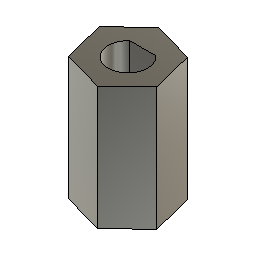
4_Assembly_Wheel - Center - Left v19 (Autodesk Fusion 360 archive; units mm, degrees)
design "Moyeu 18mm"
Autodesk Fusion 360 part; units mm, degrees
note: some values were not read from the file. Chosen so that the rebuilt part matches the saved one: a direction; which face or edge a step refers to. Set by a fixed rule: which sketch regions a step uses.
sketch "Sketch1" plane through (0, 0, 0) normal (0, 0, 1) x (1, 0, 0)
  line L0 (6.5544, -1.8584) -> (4.8866, 4.747)
  line L1 (4.8866, 4.747) -> (-1.6677, 6.6055)
  line L2 (-1.6677, 6.6055) -> (-6.5544, 1.8584)
  line L3 (-6.5544, 1.8584) -> (-4.8866, -4.747)
  line L4 (-4.8866, -4.747) -> (1.6677, -6.6055)
  line L5 (1.6677, -6.6055) -> (6.5544, -1.8584)
  circle A0 centre (0, 0) radius 5
  circle A1 centre (0, 0) radius 3.2
  line L6 (-2.1166, 2.4) -> (2.1166, 2.4)
  line L7 (0, -3.2) -> (9, -3.2) construction
  dimension "d1" = 11.8
  dimension "d2" = 10
  dimension "d7" = 6.4
  dimension "d10" = 5.6
  constraint coincident A0.centre A1.centre
  constraint coincident A1 L6.start
  constraint coincident A1 L6.end
  constraint horizontal L6
  constraint coincident A1 L7.start
  constraint tangent A1 L7
  constraint horizontal L7
  measures "d1" distance of L2 L5
  measures "d2" diameter of A0
  measures "d7" diameter of A1
  measures "d10" distance of L6 L7.start
extrude "Extrude1" add sketch "Sketch1" along normal blind 20 contours A0 | A1 L6 picked at (-0.1815, 2.7157)
extrude "Extrude2" add sketch "Sketch1" along normal blind 20 contours L0 L1 L2 L3 L4 L5

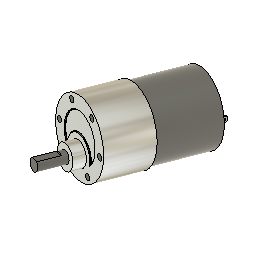
design "Moteur D37"
Autodesk Fusion 360 part; units mm, degrees
sketch "Sketch1" plane through (0, 0, 0) normal (0, 0, 1) x (1, 0, 0)
  circle A0 centre (0, 0) radius 17.4
  dimension "d2" = 34.8
  measures "d2" diameter of A0
extrude "Extrude2" add sketch "Sketch1" along normal blind 30.7
sketch "Sketch2" plane through (0, 0, 30.7) normal (0, 0, 1) x (-1, 0, 0)
  circle A0 centre (0, 0) radius 17.4
  circle A1 centre (0, 0) radius 18.4
  dimension "d7" = 36.8
  constraint coincident A0.centre A1.centre
  measures "d7" diameter of A1
extrude "Extrude3" add sketch "Sketch2" along normal blind 24 contours A0 | A1
sketch "Sketch3" plane through (0, 0, 54.7) normal (0, 0, 1) x (-1, 0, 0)
  circle A0 centre (0, 0) radius 18.4
  circle A1 centre (0, 7) radius 6
  circle A2 centre (0, 7) radius 3
  circle A3 centre (15.5, 0) radius 1.5
  circle A4 centre (7.75, -13.4234) radius 1.5
  circle A5 centre (-7.75, -13.4234) radius 1.5
  circle A6 centre (-15.5, 0) radius 1.5
  circle A7 centre (7.75, 13.4234) radius 1.5
  circle A8 centre (-7.75, 13.4234) radius 1.5
  line L0 (29.0647, 0) -> (-35.9353, 0) construction
  line L1 (7.75, 13.4234) -> (-7.75, 13.4234) construction
  line L2 (-7.75, 13.4234) -> (7.75, 13.4234) construction
  line L3 (7.75, -13.4234) -> (-7.75, -13.4234) construction
  circle A9 centre (0, 7) radius 9
  circle A10 centre (0, 0) radius 11.5
  dimension "d10" = 12
  dimension "d11" = 7
  dimension "d14" = 6
  dimension "d20" = 3
  dimension "d21" = 3
  dimension "d22" = 3
  dimension "d23" = 3
  dimension "d24" = 3
  dimension "d25" = 3
  dimension "d26" = 15.5
  dimension "d27" = 15.5
  dimension "d31" = 15.5
  dimension "d32" = 15.5
  dimension "d33" = 15.5
  dimension "d34" = 15.5
  dimension "d35" = 15.5
  dimension "d36" = 15.5
  dimension "d54" = 23
  dimension "d55" = 18
  constraint concentric A1 A2
  constraint horizontal L0
  constraint coincident A6.centre L0
  constraint coincident A0.centre L0
  constraint coincident A3.centre L0
  constraint coincident A8.centre L1.end
  constraint parallel L1 L2
  constraint coincident A7.centre L1.start
  constraint coincident A4.centre L3.start
  constraint coincident A5.centre L3.end
  constraint parallel L0 L1
  constraint parallel L0 L3
  constraint concentric A2 A9
  constraint coincident A0.centre A10.centre
  measures "d10" diameter of A1
  measures "d11" distance of A1.centre A0.centre
  measures "d14" diameter of A2
  measures "d20" diameter of A3
  measures "d21" diameter of A4
  measures "d22" diameter of A5
  measures "d23" diameter of A6
  measures "d24" diameter of A7
  measures "d25" diameter of A8
  measures "d26" distance of A0.centre A6.centre
  measures "d27" distance of A0.centre A3.centre
  measures "d31" distance of A3.centre A7.centre
  measures "d32" distance of A6.centre A8.centre
  measures "d33" distance of A7.centre A8.centre
  measures "d34" distance of A3.centre A4.centre
  measures "d35" distance of A5.centre A6.centre
  measures "d36" distance of A4.centre A5.centre
  measures "d54" diameter of A10
  measures "d55" diameter of A9
extrude "Extrude4" add sketch "Sketch3" along normal blind 6 contours A1 A10 | A1 A10 | A2
extrude "Extrude5" add sketch "Sketch3" along normal blind 20 contours A2
extrude "Extrude11" cut sketch "Sketch3" against normal blind 0.5 contours A9 A10
sketch "Sketch5" plane through (0, 0, 74.7) normal (0, 0, 1) x (-1, 0, 0)
  circle A0 centre (0, 7) radius 3
  line L0 (6, 2) -> (-6, 2)
  line L1 (-6, 2) -> (-6, 4.6)
  line L2 (-6, 4.6) -> (6, 4.6)
  line L3 (6, 4.6) -> (6, 2)
  line L4 (9, 10) -> (-8, 10) construction
  circle A1 centre (0, 7) radius 3
  dimension "d17" = 5.4
  constraint horizontal L0
  constraint vertical L1
  constraint horizontal L2
  constraint vertical L3
  constraint perpendicular L3 L4
  constraint tangent L4 A1
  measures "d17" distance of L2 L4
extrude "Extrude6" cut sketch "Sketch5" against normal blind 11 contours A0 L2 A1 picked at (0.4799, 4.5227)
extrude "Extrude7" cut sketch "Sketch3" against normal blind 10 contours A7 A9 | A7 A9 | A8 A9 | A8 A9 | A3 | A4 | A5 | A6
sketch "Sketch6" plane through (0, 0, 0) normal (0, 0, -1) x (1, 0, 0)
  circle A0 centre (0, 0) radius 17.4
  line L0 (-11.25, 0) -> (11.25, 0)
  line L1 (-11, -1.45) -> (-11.5, -1.45)
  line L2 (-11.5, -1.45) -> (-11.5, 1.45)
  line L3 (-11.5, 1.45) -> (-11, 1.45)
  line L4 (-11, 1.45) -> (-11, -1.45)
  line L5 (-11, -1.45) -> (-11.5, 1.45) construction
  line L6 (-11.5, -1.45) -> (-11, 1.45) construction
  line L7 (11.5, -1.45) -> (11, -1.45)
  line L8 (11, -1.45) -> (11, 1.45)
  line L9 (11, 1.45) -> (11.5, 1.45)
  line L10 (11.5, 1.45) -> (11.5, -1.45)
  line L11 (11.5, -1.45) -> (11, 1.45) construction
  line L12 (11, -1.45) -> (11.5, 1.45) construction
  circle A1 centre (-11.25, 0) radius 2.5
  circle A2 centre (11.25, 0) radius 2.5
  point P0 (-11.25, 0)
  point P1 (11.25, 0)
  dimension "d39" = 22.5
  dimension "d40" = 2.9
  dimension "d41" = 0.5
  dimension "d42" = 2.9
  dimension "d43" = 0.5
  dimension "d50" = 5
  dimension "d51" = 5
  constraint horizontal L0
  constraint midpoint A0.centre L0
  constraint perpendicular L1 L2
  constraint parallel L1 L3
  constraint parallel L2 L4
  constraint horizontal L1
  constraint coincident L5 P0
  constraint coincident L6 P0
  constraint coincident P0 L0.start
  constraint perpendicular L7 L8
  constraint parallel L7 L9
  constraint parallel L8 L10
  constraint horizontal L7
  constraint coincident L11 P1
  constraint coincident L12 P1
  constraint coincident P1 L0.end
  measures "d39" distance of P0 P1
  measures "d40" distance of L1.end L2.end
  measures "d41" distance of L2.end L3.end
  measures "d42" distance of L7.end L8.end
  measures "d43" distance of L8.end L9.end
  measures "d50" diameter of A1
  measures "d51" diameter of A2
extrude "Extrude8" add sketch "Sketch6" along normal blind 5 contours L1 L2 L3 L4 | L7 L8 L9 L10
extrude "Extrude10" add sketch "Sketch6" along normal blind 0.1 contours A1 | A2
sketch "Sketch7" plane through (-11.5, 0, 0) normal (-1, 0, 0) x (0, -1, 0)
  line L0 (-1.45, -0.1) -> (-1.45, -5)
  line L1 (-1.45, -5) -> (1.45, -5)
  line L2 (1.45, -5) -> (1.45, -0.1)
  line L3 (-0.5019, -3.25) -> (-0.5019, -3.75)
  arc A0 (-0.5019, -3.75) -> (0.5019, -3.75) centre (0, -3.75) ccw
  line L4 (0.5019, -3.75) -> (0.5019, -3.25)
  arc A1 (0.5019, -3.25) -> (-0.5019, -3.25) centre (0, -3.25) ccw
  line L5 (0, -3.25) -> (0, -3.75) construction
  line L6 (1.45, -0.1) -> (-1.45, -0.1)
  point P0 (0, -3.5)
  point P1 (0, -5)
  dimension "d46" = 0.5
  dimension "d47" = 1.5
  constraint tangent L3 A0
  constraint tangent A0 L4
  constraint parallel L3 L4
  constraint tangent L4 A1
  constraint tangent L3 A1
  constraint vertical L5
  constraint midpoint L5 P0
  constraint midpoint L1 P1
  measures "d46" distance of A1.centre A0.centre
  measures "d47" distance of P0 P1
extrude "Extrude9" cut sketch "Sketch7" against normal through all contours L3 A0 L4 A1
fillet "Fillet1" radius 1 4 edges at (-11.25, -1.45, -5) (-11.25, 1.45, -5) (11.25, 1.45, -5) (11.25, -1.45, -5)
fillet "Fillet2" radius 0.3 2 edges at (0, 11.5, 54.7) (0, 2, 54.7)
move_body "Move1" bodies 1 to x (0.965926, -0.257834, 0.022558) y (0, 0.087156, 0.996195) z (-0.258819, -0.96225, 0.084186) at (7.9457, 29.5411, 28.1155)
